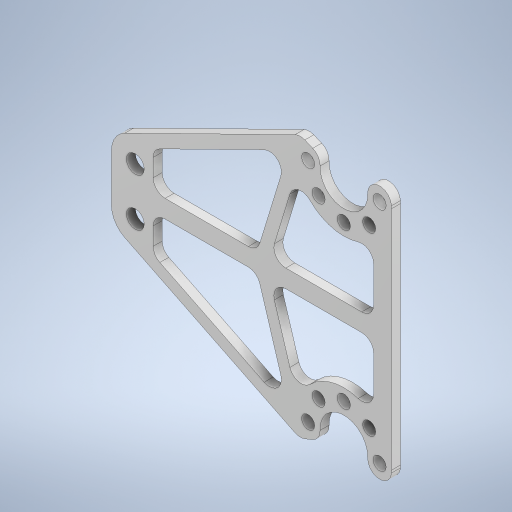
# Autodesk Inventor part: シン・膝
Saved by Autodesk Inventor 2024 (Build 280153000, 153)
## iProperties
Created: 2023-11-03
Part Number: シン・膝
Material: アルミニウム 2014-T4
Document SubType Name: Modeling
Designer: right
Density: 2.8 g/cm^3
Appearance: サテン
Author: right
Autodesk Inventor part; units mm, degrees
ref_plane "YZ Plane" through (0, 0, 0) normal (1, 0, 0) x (0, 1, 0)
ref_plane "XZ Plane" through (0, 0, 0) normal (0, 1, 0) x (-1, 0, 0)
ref_plane "XY Plane" through (0, 0, 0) normal (0, 0, 1) x (1, 0, 0)
sketch "スケッチ1" plane through (0, 0, 0) normal (0, 0, 1) x (1, 0, 0)
  circle A0 centre (17.5, 19) radius 4
  circle A1 centre (-17.5, 4) radius 1.5
  line L0 (-17.508, 0) -> (0, 0) construction
  circle A2 centre (17.5, 19) radius 6 construction
  circle A3 centre (17.5, 25) radius 1.1
  circle A4 centre (13.2574, 23.2426) radius 1.1
  circle A5 centre (11.5, 19) radius 1.1
  circle A6 centre (13.2574, 14.7574) radius 1.1
  circle A7 centre (17.5, 13) radius 1.1
  circle A8 centre (21.7426, 14.7574) radius 1.1
  circle A9 centre (23.5, 19) radius 1.1
  circle A10 centre (21.7426, 23.2426) radius 1.1
  circle A11 centre (17.5, -19) radius 4
  circle A12 centre (17.5, -19) radius 6 construction
  circle A13 centre (17.5, -25) radius 1.1
  circle A14 centre (13.2574, -23.2426) radius 1.1
  circle A15 centre (11.5, -19) radius 1.1
  circle A16 centre (13.2574, -14.7574) radius 1.1
  circle A17 centre (17.5, -13) radius 1.1
  circle A18 centre (21.7426, -14.7574) radius 1.1
  circle A19 centre (23.5, -19) radius 1.1
  circle A20 centre (21.7426, -23.2426) radius 1.1
  circle A21 centre (17.5, 19) radius 8
  line L1 (13.2574, 23.2426) -> (11.5, 19) construction
  line L2 (21.7426, 23.2426) -> (23.5, 19) construction
  line L3 (17.5, 19) -> (24.891, 22.0615)
  line L4 (17.5, 25) -> (17.5, 19) construction
  line L5 (17.5, 19) -> (10.109, 22.0615)
  line L6 (10.109, 22.0615) -> (-19.2678, 7.5882)
  line L7 (10.109, -22.0615) -> (-19.2678, -7.5882)
  circle A22 centre (17.5, -19) radius 8
  line L8 (17.5, -19) -> (24.891, -22.0615)
  line L9 (17.5, -19) -> (10.109, -22.0615)
  circle A23 centre (-17.5, 4) radius 4
  circle A24 centre (-17.5, -4) radius 1.5
  circle A25 centre (-17.5, -4) radius 4
  line L10 (-21.5, 4) -> (-21.5, -4)
  line L11 (25.5, 19) -> (25.5, -19)
  point P0 (22.6213, 21.1213)
  point P1 (25, 0)
  point P2 (21.1955, 20.5307)
  point P3 (13.8045, 20.5307)
  point P4 (13.8045, -20.5307)
  point P5 (21.1955, -20.5307)
  point P6 (-19.2678, 7.5882)
  dimension "d24" = 8
  dimension "d0" = 8
  dimension "d1" = 3
  dimension "d2" = 35
  dimension "d3" = 15
  dimension "d4" = 17.5
  dimension "d5" = 12
  dimension "d6" = 2.2
  dimension "d9" = 360
  dimension "d11" = 16
  constraints: 24 centre point, 24 end point, 17 symmetric about line, 8 point on circle, 5 coincident, 3 tangent, 2 horizontal, 2 horizontal alignment, 2 vertical, 2 vertical alignment, 1 midpoint, 1 point on line, 35 other
  measures "d0" diameter of A0
  measures "d1" diameter of A1
  measures "d2" horizontal distance of A0.centre A1.centre
  measures "d3" vertical distance of A0.centre A1.centre
  measures "d4" horizontal distance of L0.end A0.centre
  measures "d5" diameter of A2
  measures "d6" diameter of A3
  measures "d11" diameter of A21
extrude "押し出し1" add sketch "スケッチ1" along normal blind 1.5 contours A0 L3 A21 L5 | A21 L11 A22 L7 A25 A23 L6 | A23 | A22 L8 A11 L9 | A23 A25 L10 | A25 picked at (20.0269, 12.879) picked at (20.0269, -12.879)
fillet "フィレット1" radius 2 8 edges at (24.891, 22.0615, 0.75) (21.1955, 20.5307, 0.75) (13.8045, 20.5307, 0.75) (10.109, 22.0615, 0.75) (24.891, -22.0615, 0.75) (21.1955, -20.5307, 0.75) (13.8045, -20.5307, 0.75) (10.109, -22.0615, 0.75)
sketch "スケッチ2" plane through (0, 0, 1.5) normal (0, 0, 1) x (1, 0, 0)
  arc A0 (9.2965, -21.6612) -> (10.9458, -21.7149) centre (10.1804, -19.8671) ccw projected
  line L0 (10.9458, -21.7149) -> (12.2737, -21.1648) projected
  arc A1 (12.2737, -21.1648) -> (13.5056, -19.2114) centre (11.5084, -19.317) ccw projected
  arc A2 (21.4944, -19.2114) -> (13.5056, -19.2114) centre (17.5, -19) ccw projected
  arc A3 (21.4944, -19.2114) -> (25.4888, -19.4227) centre (23.4916, -19.317) ccw projected
  arc A4 (25.4888, -19.4227) -> (25.5, -19) centre (17.5, -19) ccw projected
  line L1 (25.5, -19) -> (25.5, 19) projected
  arc A5 (25.5, 19) -> (25.4888, 19.4227) centre (17.5, 19) ccw projected
  arc A6 (25.4888, 19.4227) -> (21.4944, 19.2114) centre (23.4916, 19.317) ccw projected
  arc A7 (13.5056, 19.2114) -> (21.4944, 19.2114) centre (17.5, 19) ccw projected
  arc A8 (13.5056, 19.2114) -> (12.2737, 21.1648) centre (11.5084, 19.317) ccw projected
  line L2 (12.2737, 21.1648) -> (10.9458, 21.7149) projected
  arc A9 (10.9458, 21.7149) -> (9.2965, 21.6612) centre (10.1804, 19.8671) ccw projected
  line L3 (9.2965, 21.6612) -> (-19.2678, 7.5882) projected
  arc A10 (-19.2678, 7.5882) -> (-21.5, 4) centre (-17.5, 4) ccw projected
  line L4 (-21.5, 4) -> (-21.5, -4) projected
  arc A11 (-21.5, -4) -> (-19.2678, -7.5882) centre (-17.5, -4) ccw projected
  line L5 (-19.2678, -7.5882) -> (9.2965, -21.6612) projected
  circle A12 centre (11.5, -19) radius 1.1 projected
  circle A13 centre (13.2574, -14.7574) radius 1.1 projected
  circle A14 centre (17.5, -13) radius 1.1 projected
  circle A15 centre (21.7426, -14.7574) radius 1.1 projected
  circle A16 centre (23.5, -19) radius 1.1 projected
  circle A17 centre (-17.5, -4) radius 1.5 projected
  circle A18 centre (-17.5, 4) radius 1.5 projected
  circle A19 centre (11.5, 19) radius 1.1 projected
  circle A20 centre (13.2574, 14.7574) radius 1.1 projected
  circle A21 centre (17.5, 13) radius 1.1 projected
  circle A22 centre (21.7426, 14.7574) radius 1.1 projected
  circle A23 centre (23.5, 19) radius 1.1 projected
  line L6 (9.5183, 19.5409) -> (-14.5, 7.7076)
  line L7 (9.2965, 21.6612) -> (-19.2678, 7.5882) projected
  circle A24 centre (17.5, 19) radius 8
  line L8 (-14.5, 7.7076) -> (-14.5, 0)
  line L9 (-14.5, 0) -> (0, 0) construction
  line L10 (9.5183, -19.5409) -> (-14.5, -7.7076)
  circle A25 centre (17.5, -19) radius 8
  line L11 (-14.5, -7.7076) -> (-14.5, 0)
  line L12 (22.5, 12.755) -> (22.5, -12.755)
  line L13 (25.5, -19) -> (25.5, 19) construction
  line L14 (-14.5, 1.5) -> (22.5, 1.5)
  line L15 (22.5, 1.5) -> (22.5, -1.5)
  line L16 (22.5, -1.5) -> (-14.5, -1.5)
  line L17 (-14.5, -1.5) -> (-14.5, 1.5)
  line L18 (9.5183, 19.5409) -> (4, 1.5) construction
  line L19 (8.287, 18.9343) -> (2.9543, 1.5)
  line L20 (9.7692, 16.9423) -> (5.0457, 1.5)
  line L21 (8.287, -18.9343) -> (2.9543, -1.5)
  line L22 (9.7692, -16.9423) -> (5.0457, -1.5)
  point P0 (22.5, 0)
  point P1 (10.1995, 18.3493)
  point P2 (4.8668, 0.915)
  point P3 (2.9543, -1.5)
  point P4 (5.0457, -1.5)
  dimension "d25" = 2
  dimension "d26" = 3
  dimension "d27" = 3
  dimension "d28" = 3
  dimension "d29" = 1
  dimension "d30" = 1
  constraints: 30 end point, 9 symmetric about line, 6 point on circle, 5 parallel, 5 point on line, 3 horizontal alignment, 3 midpoint, 2 centre point, 2 horizontal, 1 coincident, 1 perpendicular, 1 vertical, 1 other
  measures "d25" distance between parallel lines of L3 L6
  measures "d26" horizontal distance of A18.centre L6.end
  measures "d27" distance between parallel lines of L1 L12
  measures "d28" distance between parallel lines of L16 L14
  measures "d29" distance between parallel lines of L18 L19
  measures "d30" distance between parallel lines of L18 L20
extrude "押し出し2" cut sketch "スケッチ2" against normal blind 1.5 contours L10 L11 L16 L21 | L22 L16 L12 A25 | L12 L14 L20 A24 | L8 L6 L19 L14
fillet "フィレット2" radius 2 16 edges at (9.7692, -16.9423, 0.75) (8.287, -18.9343, 0.75) (22.5, -12.755, 0.75) (22.5, -1.5, 0.75) (5.0457, -1.5, 0.75) (5.0457, 1.5, 0.75) (22.5, 1.5, 0.75) (9.7692, 16.9423, 0.75) (22.5, 12.755, 0.75) (2.9543, -1.5, 0.75) (2.9543, 1.5, 0.75) (-14.5, 1.5, 0.75) (-14.5, 7.7076, 0.75) (8.287, 18.9343, 0.75) (-14.5, -7.7076, 0.75) (-14.5, -1.5, 0.75)
equation "\"d4\" = 0.5 * d2"
equation "\"d30\" = d29"
